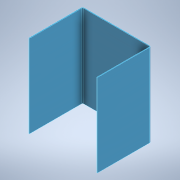
# Autodesk Inventor part: SuportHdd_GoleaCristian
Saved by Autodesk Inventor 2021 (Build 250183000, 183)
## iProperties
Created: 2021-05-17
Part Number: SuportHdd_GoleaCristian
Material: Steel, Mild
Document SubType Name: Sheet Metal
Designer: Crist
Density: 7.85 g/cm^3
Sheet Metal Rule: Default_mm
Appearance: Sky Blue Dark
Author: Crist
Autodesk Inventor part; units mm, degrees
ref_plane "YZ Plane" through (0, 0, 0) normal (1, 0, 0) x (0, 1, 0)
ref_plane "XZ Plane" through (0, 0, 0) normal (0, 1, 0) x (-1, 0, 0)
ref_plane "XY Plane" through (0, 0, 0) normal (0, 0, 1) x (1, 0, 0)
sketch "Sketch1" plane through (0, 0, 0) normal (0, 0, 1) x (1, 0, 0)
  line L0 (-51, 61.5) -> (51, 61.5)
  line L1 (51, 61.5) -> (51, -61.5)
  line L2 (51, -61.5) -> (-51, -61.5)
  line L3 (-51, -61.5) -> (-51, 61.5)
  point P0 (0, 0)
  dimension "d0" = 102
  dimension "d1" = 123
  dimension "d2" = 61.5
  dimension "d3" = 51
  measures "d0" distance of L1.end L2.end
  measures "d1" distance of L0.end L1.end
  measures "d2" distance from line of point (0, 0) L0
  measures "d3" distance from line of L3 point (0, 0)
extrude "Plate1" add sketch "Sketch1" along normal blind 1
sketch "Sketch2" plane through (-50, -61.5, 0) normal (-1, 0, 0) x (0, -1, 0)
  line L0 (-123, 0) -> (0, 0)
  line L1 (0, 0) -> (0, 80)
  line L2 (0, 80) -> (-123, 80)
  line L3 (-123, 80) -> (-123, 0)
  constraints: 6 end point, 1 horizontal, 1 perpendicular, 1 vertical
edge flange "Flange1" height 80 angle 90 thickness 1 bend radius 1 thickness toward (-1, 0, 0) relief straight relief width 1 relief depth 0.5 corner gap 1 corner form 0 edges at (-51, 0, 1) (51, 0, 1) wall of the first edge with corners at (-50, 61.5, 0) (-50, -61.5, 0) (-50, -61.5, 80) (-50, 61.5, 80)
bend "Bend1"
corner "Corner1"
equation "\"d4\" = Thickness"
equation "\"d5\" = BendReliefWidth"
equation "\"d6\" = BendReliefDepth"
equation "\"d7\" = MinimumRemnant"
equation "\"d8\" = TransitionRadius"
equation "\"d11\" = BendRadius"
equation "\"d12\" = CornerReliefSize"
equation "\"d13\" = GapSize"
equation "\"d14\" = JacobiRadiusSize"
equation "\"d2\" = 0.5 * d1"
equation "\"d3\" = 0.5 * d0"
equation "\"BendRadius\" = Thickness"
equation "\"BendReliefWidth\" = Thickness"
equation "\"BendReliefDepth\" = 0.5 * Thickness"
equation "\"CornerReliefSize\" = 4 * Thickness"
equation "\"MinimumRemnant\" = 2 * Thickness"
equation "\"TransitionRadius\" = BendRadius"
equation "\"JacobiRadiusSize\" = BendRadius"
equation "\"GapSize\" = Thickness"
equation "\"Thickness\" = 1"
body "Solid1"
